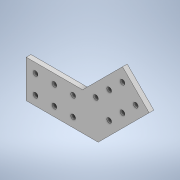
# Autodesk Inventor part: 2x3 Vplate
Saved by Autodesk Inventor 2020 (Build 240168000, 168)
## iProperties
Created: 2020-01-28
Part Number: 2x3 Vplate
Material: Generic
Document SubType Name: Modeling
Designer: 339294
Density: 1 g/cm^3
Appearance: Default
Author: 339294
Autodesk Inventor part; units mm, degrees
ref_plane "YZ Plane" through (0, 0, 0) normal (1, 0, 0) x (0, 1, 0)
ref_plane "XZ Plane" through (0, 0, 0) normal (0, 1, 0) x (-1, 0, 0)
ref_plane "XY Plane" through (0, 0, 0) normal (0, 0, 1) x (1, 0, 0)
sketch "Sketch1" plane through (0, 0, 0) normal (0, 0, 1) x (1, 0, 0)
  line L0 (0, 0) -> (0, 50.8)
  line L1 (0, 50.8) -> (76.2, 50.8)
  line L2 (76.2, 50.8) -> (130.0815, 104.6815)
  line L3 (130.0815, 104.6815) -> (166.0026, 68.7605)
  line L4 (166.0026, 68.7605) -> (97.242, 0)
  line L5 (97.242, 0) -> (0, 0)
  circle A0 centre (12.7, 12.7) radius 3.2512
  circle A1 centre (12.7, 38.1) radius 3.2512
  circle A2 centre (38.1, 12.7) radius 3.2512
  circle A3 centre (38.1, 38.1) radius 3.2512
  circle A4 centre (63.5, 12.7) radius 3.2512
  circle A5 centre (63.5, 38.1) radius 3.2512
  circle A6 centre (130.0815, 86.721) radius 3.2512
  circle A7 centre (112.121, 68.7605) radius 3.2512
  circle A8 centre (94.1605, 50.8) radius 3.2512
  circle A9 centre (148.042, 68.7605) radius 3.2512
  circle A10 centre (130.0815, 50.8) radius 3.2512
  circle A11 centre (112.121, 32.8395) radius 3.2512
  dimension "d0" = 50.8
  dimension "d1" = 76.2
  dimension "d2" = 76.2
  dimension "d3" = 135
  dimension "d4" = 50.8
  dimension "d5" = 6.5024
  dimension "d6" = 12.7
  dimension "d7" = 12.7
  dimension "d10" = 25.4
  dimension "d13" = 25.4
  dimension "d16" = 6.5024
  dimension "d17" = 12.7
  dimension "d18" = 12.7
  dimension "d21" = 25.4
  dimension "d24" = 25.4
  constraints: 12 centre point, 12 end point, 4 perpendicular, 2 vertical, 1 horizontal, 22 other
  measures "d0" distance of L0.start L0.end
  measures "d1" distance of L0.end L1.end
  measures "d2" distance of L1.end L2.end
  measures "d3" angle of L2 L1
  measures "d4" distance of L2.end L3.end
  measures "d5" diameter of A0
  measures "d6" distance from line of L0 A0.centre
  measures "d7" distance from line of L5 A0.centre
  measures "d10" distance of A0.centre A1.centre
  measures "d13" distance of A0.centre A2.centre
  measures "d16" diameter of A6
  measures "d17" distance from line of L2 A6.centre
  measures "d18" distance from line of L3 A6.centre
  measures "d21" distance of A6.centre A7.centre
  measures "d24" distance of A6.centre A9.centre
extrude "Extrusion1" add sketch "Sketch1" along normal blind 6.35
body "Solid1"
